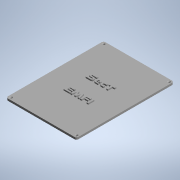
# Autodesk Inventor part: skr_case_top
Saved by Autodesk Inventor 2022 (Build 260153000, 153)
## iProperties
Part Number: skr_case_top
Material: Allgemein
Document SubType Name: Modellieren
Designer: Niclas
Appearance: Vorgabe
Author: Niclas
Autodesk Inventor part; units mm, degrees
ref_plane "YZ-Ebene" through (0, 0, 0) normal (1, 0, 0) x (0, 1, 0)
ref_plane "XZ-Ebene" through (0, 0, 0) normal (0, 1, 0) x (-1, 0, 0)
ref_plane "XY-Ebene" through (0, 0, 0) normal (0, 0, 1) x (1, 0, 0)
sketch "Skizze1" plane through (0, 0, 0) normal (0, 1, 0) x (-1, 0, 0)
  line L0 (-4, 0) -> (-136, 0)
  line L1 (-140, -4) -> (-140, -190)
  line L2 (-136, -194) -> (-4, -194)
  line L3 (0, -190) -> (0, -4)
  arc A0 (0, -4) -> (-4, 0) centre (-4, -4) ccw
  arc A1 (-4, -194) -> (0, -190) centre (-4, -190) ccw
  arc A2 (-140, -190) -> (-136, -194) centre (-136, -190) ccw
  arc A3 (-136, 0) -> (-140, -4) centre (-136, -4) ccw
  point P0 (0, 0)
  point P1 (0, 0)
  point P2 (-140, 0)
  point P3 (0, -194)
  dimension "d0" = 140
  dimension "d1" = 194
  dimension "d2" = 4
  constraints: 8 end point, 8 point on circle, 8 tangent, 6 point on line, 4 centre point, 3 equal radius, 2 parallel, 1 coincident, 1 horizontal, 1 perpendicular
  measures "d0" distance of point (0, 0) point (-140, 0)
  measures "d1" distance of point (0, -194) point (0, 0)
  measures "d2" radius of A0
extrude "Extrusion1" add sketch "Skizze1" along normal blind 4
sketch "Skizze2" plane through (0, 4, 0) normal (0, 1, 0) x (1, 0, 0)
  line L0 (140, 4) -> (140, 190) projected
  line L1 (136, 194) -> (4, 194) projected
  line L2 (4, 0) -> (136, 0) projected
  line L3 (0, 190) -> (0, 4) projected
  point P0 (0, 0)
  point P1 (135, 189)
  point P2 (5, 189)
  point P3 (5, 5)
  point P4 (135, 5)
  dimension "d21" = 20
  dimension "d5" = 5
  dimension "d6" = 5
  dimension "d7" = 5
  dimension "d8" = 5
  dimension "d9" = 5
  dimension "d10" = 5
  dimension "d11" = 5
  dimension "d12" = 5
  measures "d5" distance from line of point (135, 189) L0
  measures "d6" distance from line of L1 point (135, 189)
  measures "d7" distance from line of L0 point (135, 5)
  measures "d8" distance from line of L2 point (135, 5)
  measures "d9" distance from line of L2 point (5, 5)
  measures "d10" distance from line of L3 point (5, 5)
  measures "d11" distance from line of L3 point (5, 189)
  measures "d12" distance from line of point (5, 189) L1
hole "Bohrung1" at (135, 4, -189) at (5, 4, -189) at (5, 4, -5) at (135, 4, -5) direction (0, -1, 0) diameter 3 end through all countersink diameter 5.5 countersink angle 82
sketch "Skizze3" plane through (0, 4, 0) normal (0, 1, 0) x (1, 0, 0)
  line L0 (20, 147) -> (120, 147) construction
  line L1 (120, 147) -> (120, 47) construction
  line L2 (120, 47) -> (20, 47) construction
  line L3 (20, 47) -> (20, 147) construction
  line L4 (0, 190) -> (0, 4) projected
  line L5 (4, 0) -> (136, 0) projected
  line L6 (45.9308, 112.5631) -> (45.9308, 115.7124)
  line L7 (45.9308, 115.7124) -> (55.0274, 115.7124)
  spline S0 degree 2 poles (55.0274, 115.7124) (55.3895, 115.7124) (55.8394, 116.1403) (55.8394, 116.5353) knots 0 0 0 1 2 2 2
  spline S1 degree 2 poles (55.8394, 116.5353) (55.8394, 116.9304) (55.3895, 117.3803) (55.0274, 117.3803) knots 0 0 0 1 2 2 2
  line L8 (55.0274, 117.3803) -> (49.6726, 117.3803)
  spline S2 degree 2 poles (49.6726, 117.3803) (48.8276, 117.3803) (47.3902, 117.9179) (46.3587, 118.8726) (45.7772, 120.2223) (45.7772, 121.0452) knots 0 0 0 1 2 3 4 4 4
  spline S3 degree 2 poles (45.7772, 121.0452) (45.7772, 121.8682) (46.3587, 123.2398) (47.3902, 124.2164) (48.8276, 124.7431) (49.6726, 124.7431) knots 0 0 0 1 2 3 4 4 4
  line L9 (49.6726, 124.7431) -> (58.9228, 124.7431)
  line L10 (58.9228, 124.7431) -> (58.9228, 121.6048)
  line L11 (58.9228, 121.6048) -> (49.8262, 121.6048)
  spline S4 degree 2 poles (49.8262, 121.6048) (49.4641, 121.6048) (49.0361, 121.1988) (49.0361, 120.8038) knots 0 0 0 1 2 2 2
  spline S5 degree 2 poles (49.0361, 120.8038) (49.0361, 120.4307) (49.4641, 119.9808) (49.8262, 119.9808) knots 0 0 0 1 2 2 2
  line L12 (49.8262, 119.9808) -> (55.181, 119.9808)
  spline S6 degree 2 poles (55.181, 119.9808) (56.0369, 119.9808) (57.4634, 119.4322) (58.5168, 118.4666) (59.0984, 117.095) (59.0984, 116.2939) knots 0 0 0 1 2 3 4 4 4
  spline S7 degree 2 poles (59.0984, 116.2939) (59.0984, 115.449) (58.5168, 114.0774) (57.4634, 113.0898) (56.0369, 112.5631) (55.181, 112.5631) knots 0 0 0 1 2 3 4 4 4
  line L13 (55.181, 112.5631) -> (45.9308, 112.5631)
  spline S8 degree 2 poles (65.2322, 112.5631) (64.1459, 112.5631) (62.3134, 113.2325) (60.9638, 114.4724) (60.2176, 116.1952) (60.2176, 117.2486) knots 0 0 0 1 2 3 4 4 4
  spline S9 degree 2 poles (60.2176, 117.2486) (60.2176, 118.28) (60.9638, 120.0028) (62.3134, 121.2318) (64.1459, 121.9121) (65.2322, 121.9121) knots 0 0 0 1 2 3 4 4 4
  line L14 (65.2322, 121.9121) -> (67.6134, 121.9121)
  spline S10 degree 2 poles (67.6134, 121.9121) (68.4144, 121.9121) (69.6105, 121.4622) (70.4225, 120.6721) (70.8175, 119.5639) (70.8175, 118.9165) knots 0 0 0 1 2 3 4 4 4
  spline S11 degree 2 poles (70.8175, 118.9165) (70.8175, 117.6765) (69.391, 116.4366) (67.756, 116.4366) knots 0 0 0 1 2 2 2
  line L15 (67.756, 116.4366) -> (64.4312, 116.4366)
  line L16 (64.4312, 116.4366) -> (64.4312, 118.1484)
  line L17 (64.4312, 118.1484) -> (67.1086, 118.1484)
  spline S12 degree 2 poles (67.1086, 118.1484) (67.8328, 118.1484) (67.8328, 118.7958) knots 0 0 0 1 1 1
  spline S13 degree 2 poles (67.8328, 118.7958) (67.8328, 119.498) (67.1196, 119.498) knots 0 0 0 1 1 1
  line L18 (67.1196, 119.498) -> (65.2103, 119.498)
  spline S14 degree 2 poles (65.2103, 119.498) (64.3654, 119.498) (63.3229, 118.3349) (63.3229, 117.2595) knots 0 0 0 1 2 2 2
  spline S15 degree 2 poles (63.3229, 117.2595) (63.3229, 116.1952) (64.3654, 115.1308) (65.2103, 115.1308) knots 0 0 0 1 2 2 2
  line L19 (65.2103, 115.1308) -> (70.3127, 115.1308)
  line L20 (70.3127, 115.1308) -> (70.3127, 112.5631)
  line L21 (70.3127, 112.5631) -> (65.2322, 112.5631)
  spline S16 degree 2 poles (76.9185, 112.5631) (75.8321, 112.5631) (73.9996, 113.2325) (72.65, 114.4724) (71.9038, 116.1952) (71.9038, 117.2486) knots 0 0 0 1 2 3 4 4 4
  spline S17 degree 2 poles (71.9038, 117.2486) (71.9038, 118.28) (72.65, 120.0028) (73.9996, 121.2318) (75.8321, 121.9121) (76.9185, 121.9121) knots 0 0 0 1 2 3 4 4 4
  line L22 (76.9185, 121.9121) -> (81.1321, 121.9121)
  line L23 (81.1321, 121.9121) -> (81.1321, 119.0591)
  line L24 (81.1321, 119.0591) -> (76.8965, 119.0591)
  spline S18 degree 2 poles (76.8965, 119.0591) (76.0516, 119.0591) (75.0092, 118.0715) (75.0092, 117.2486) knots 0 0 0 1 2 2 2
  spline S19 degree 2 poles (75.0092, 117.2486) (75.0092, 116.4256) (76.0516, 115.4051) (76.8965, 115.4051) knots 0 0 0 1 2 2 2
  line L25 (76.8965, 115.4051) -> (81.1321, 115.4051)
  line L26 (81.1321, 115.4051) -> (81.1321, 112.5631)
  line L27 (81.1321, 112.5631) -> (76.9185, 112.5631)
  line L28 (86.6734, 112.5631) -> (86.6734, 121.6048)
  line L29 (86.6734, 121.6048) -> (82.1965, 121.6048)
  line L30 (82.1965, 121.6048) -> (82.1965, 124.7431)
  line L31 (82.1965, 124.7431) -> (94.4313, 124.7431)
  line L32 (94.4313, 124.7431) -> (94.4313, 121.6048)
  line L33 (94.4313, 121.6048) -> (89.9544, 121.6048)
  line L34 (89.9544, 121.6048) -> (89.9544, 112.5631)
  line L35 (89.9544, 112.5631) -> (86.6734, 112.5631)
  line L36 (45.5632, 69.2569) -> (45.5632, 81.4369)
  line L37 (45.5632, 81.4369) -> (57.2494, 81.4369)
  line L38 (57.2494, 81.4369) -> (57.2494, 78.2986)
  line L39 (57.2494, 78.2986) -> (48.8441, 78.2986)
  line L40 (48.8441, 78.2986) -> (48.8441, 72.4061)
  line L41 (48.8441, 72.4061) -> (57.2714, 72.4061)
  line L42 (57.2714, 72.4061) -> (57.2714, 69.2569)
  line L43 (57.2714, 69.2569) -> (45.5632, 69.2569)
  line L44 (49.9304, 74.074) -> (49.9304, 76.6746)
  line L45 (49.9304, 76.6746) -> (57.1177, 76.6746)
  line L46 (57.1177, 76.6746) -> (57.1177, 74.074)
  line L47 (57.1177, 74.074) -> (49.9304, 74.074)
  line L48 (73.5223, 69.2569) -> (71.7337, 77.0916)
  line L49 (71.7337, 77.0916) -> (69.6159, 70.42)
  spline S20 degree 2 poles (69.6159, 70.42) (69.2758, 69.2569) (68.0797, 69.2569) knots 0 0 0 1 1 1
  line L50 (68.0797, 69.2569) -> (67.0812, 69.2569)
  spline S21 degree 2 poles (67.0812, 69.2569) (65.8851, 69.2569) (65.545, 70.42) knots 0 0 0 1 1 1
  line L51 (65.545, 70.42) -> (63.4272, 77.2123)
  line L52 (63.4272, 77.2123) -> (61.6386, 69.2569)
  line L53 (61.6386, 69.2569) -> (58.3906, 69.2569)
  line L54 (58.3906, 69.2569) -> (60.8705, 80.0433)
  spline S22 degree 2 poles (60.8705, 80.0433) (61.0131, 80.8114) (61.8361, 81.4369) (62.4616, 81.4369) knots 0 0 0 1 2 2 2
  line L55 (62.4616, 81.4369) -> (63.8222, 81.4369)
  spline S23 degree 2 poles (63.8222, 81.4369) (65.0183, 81.4369) (65.3804, 80.2518) knots 0 0 0 1 1 1
  line L56 (65.3804, 80.2518) -> (67.5859, 72.9657)
  line L57 (67.5859, 72.9657) -> (69.7805, 80.2518)
  spline S24 degree 2 poles (69.7805, 80.2518) (70.1317, 81.4369) (71.3168, 81.4369) knots 0 0 0 1 1 1
  line L58 (71.3168, 81.4369) -> (72.6884, 81.4369)
  spline S25 degree 2 poles (72.6884, 81.4369) (73.3029, 81.4369) (74.1258, 80.8114) (74.2904, 80.0433) knots 0 0 0 1 2 2 2
  line L59 (74.2904, 80.0433) -> (76.7813, 69.2569)
  line L60 (76.7813, 69.2569) -> (73.5223, 69.2569)
  line L61 (78.0432, 69.2569) -> (78.0432, 81.4369)
  line L62 (78.0432, 81.4369) -> (89.3892, 81.4369)
  line L63 (89.3892, 81.4369) -> (89.3892, 78.2986)
  line L64 (89.3892, 78.2986) -> (81.3241, 78.2986)
  line L65 (81.3241, 78.2986) -> (81.3241, 69.2569)
  line L66 (81.3241, 69.2569) -> (78.0432, 69.2569)
  line L67 (82.4104, 73.8985) -> (82.4104, 76.6527)
  line L68 (82.4104, 76.6527) -> (89.2795, 76.6527)
  line L69 (89.2795, 76.6527) -> (89.2795, 73.8985)
  line L70 (89.2795, 73.8985) -> (82.4104, 73.8985)
  line L71 (91.1669, 69.2569) -> (91.1669, 81.4369)
  line L72 (91.1669, 81.4369) -> (94.4478, 81.4369)
  line L73 (94.4478, 81.4369) -> (94.4478, 69.2569)
  line L74 (94.4478, 69.2569) -> (91.1669, 69.2569)
  point P0 (0, 0)
  dimension "d20" = 100
  dimension "d21" = 20
  dimension "d22" = 100
  dimension "d23" = 47
  constraints: 2 other
  measures "d20" distance of L0.start L0.end
  measures "d21" distance between parallel lines of L4 L3
  measures "d22" distance between parallel lines of L2 L0
  measures "d23" distance between parallel lines of L5 L2
extrude "Extrusion2" add sketch "Skizze3" along normal blind 2.5
